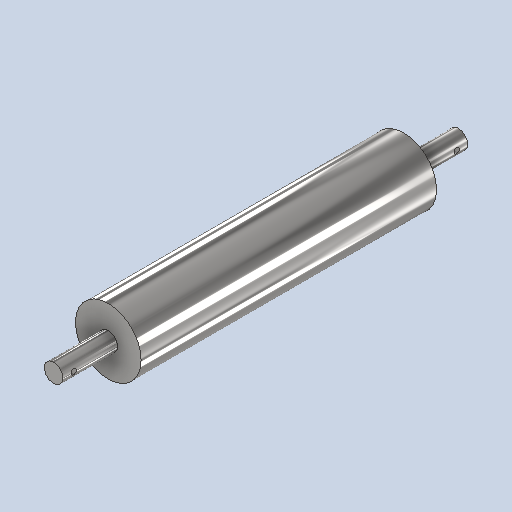
# Autodesk Inventor part: HCMUTE-CDT23-TRUC_CANG
Saved by Autodesk Inventor 2023 (Build 270158000, 158)
## iProperties
Created: 2023-10-08
Part Number: HCMUTE-CDT23-TRUC_CANG
Material: Stainless Steel
Document SubType Name: Modeling
Designer: havie
Density: 8 g/cm^3
Appearance: Steel - Polished
Author: havie
Autodesk Inventor part; units mm, degrees
ref_plane "YZ Plane" through (0, 0, 0) normal (1, 0, 0) x (0, 1, 0)
ref_plane "XZ Plane" through (0, 0, 0) normal (0, 1, 0) x (-1, 0, 0)
sketch "Sketch1" plane through (0, 0, 0) normal (0, 1, 0) x (-1, 0, 0)
  circle A0 centre (0, 0) radius 30
  dimension "d0" = 60
  constraints: 1 centre point, 1 coincident
  measures "d0" diameter of A0
extrude "Extrusion1" add sketch "Sketch1" along normal mid plane 270
sketch "Sketch2" plane through (0, -135, 0) normal (0, -1, 0) x (1, 0, 0)
  circle A0 centre (0, 0) radius 8.5
  dimension "d3" = 17
  constraints: 1 centre point, 1 coincident
  measures "d3" diameter of A0
extrude "Extrusion2" add sketch "Sketch2" along normal blind 50
sketch "Sketch3" plane through (0, 135, 0) normal (0, 1, 0) x (1, 0, 0)
  circle A0 centre (0, 0) radius 8.5 projected
  circle A1 centre (0, 0) radius 8.5
  dimension "d6" = 17
  constraints: 1 centre point, 1 coincident
  measures "d6" diameter of A1
extrude "Extrusion3" add sketch "Sketch3" along normal blind 50
ref_plane "Work Plane1" through (-9, 135, 0) normal (-1, 0, 0) x (0, 1, 0)
sketch "Sketch4" plane through (-9, 135, 0) normal (-1, 0, 0) x (0, 1, 0)
  circle A0 centre (40, 0) radius 4 projected
  circle A1 centre (-310, 0) radius 4 projected
  point P0 (-135, 0)
  constraints: 2 coincident
hole "Hole1" at (-9, 175, 0) at (-9, -175, 0) direction (1, 0, 0) diameter 4.917 end through all thread size "M6x1" class "6H" standard "ISO Metric profile"
body "Solid1"
